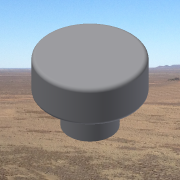
# Autodesk Inventor part: chimney
Saved by Autodesk Inventor 2014 SP1 (Build 180222100, 222)
## iProperties
Created: 2014-05-23
Part Number: chimney
Material: Generic
Document SubType Name: Modeling
Designer: Dave
Density: 1 g/cm^3
Appearance: Default
Author: Dave
Autodesk Inventor part; units mm, degrees
ref_plane "YZ Plane" through (0, 0, 0) normal (1, 0, 0) x (0, 1, 0)
ref_plane "XZ Plane" through (0, 0, 0) normal (0, 1, 0) x (-1, 0, 0)
ref_plane "XY Plane" through (0, 0, 0) normal (0, 0, 1) x (1, 0, 0)
sketch "Sketch1" plane through (0, 0, 0) normal (0, 1, 0) x (-1, 0, 0)
  circle A0 centre (0, 0) radius 127
  circle A1 centre (0, 0) radius 125.73
  dimension "d0" = 254
  dimension "d1" = 1.27
  constraints: 2 centre point, 1 coincident
  measures "d0" diameter of A0
  measures "d1" radial gap between concentric circles of A1 A0
extrude "Extrusion1" add sketch "Sketch1" along normal blind 203.2
sketch "Sketch2" plane through (0, 203.2, 0) normal (0, 1, 0) x (1, 0, 0)
  circle A0 centre (0, 0) radius 125.73 projected
  circle A1 centre (0, 0) radius 127 projected
  point P0 (0, 127)
  constraints: 1 vertical alignment, 1 other
ref_plane "Work Plane1" through (0, 203.2, -127) normal (0, 0, -1) x (-1, 0, 0)
sketch "Sketch3" plane through (0, 203.2, -127) normal (0, 0, -1) x (-1, 0, 0)
  line L0 (-6.3336, -31.75) -> (6.3664, -31.75)
  line L1 (6.3664, -31.75) -> (6.3664, -12.7)
  line L2 (6.3664, -12.7) -> (-6.3336, -12.7)
  line L3 (-6.3336, -12.7) -> (-6.3336, -31.75)
  line L4 (127, 0) -> (-127, 0) projected
  point P0 (0, -203.2)
  point P1 (0.0164, -12.7)
  dimension "d4" = 12.7
  dimension "d5" = 19.05
  dimension "d6" = 12.7
  constraints: 8 end point, 2 parallel, 1 horizontal, 1 midpoint, 1 perpendicular
  measures "d4" distance of L0.start L0.end
  measures "d5" distance of L2.end L0.start
  measures "d6" distance between parallel lines of L2 L4
extrude "Extrusion2" add sketch "Sketch3" along normal blind 1.27
sketch "Sketch4" plane through (0, 203.2, -128.27) normal (0, 0, -1) x (-1, 0, 0)
  line L0 (-6.3336, -31.75) -> (6.3664, -31.75) projected
  line L1 (6.3664, -31.75) -> (6.3664, -12.7) projected
  line L2 (-6.3336, -31.75) -> (6.3664, -31.75)
  line L3 (6.3664, -31.75) -> (6.3664, -30.48)
  line L4 (6.3664, -30.48) -> (-6.3336, -30.48)
  line L5 (-6.3336, -30.48) -> (-6.3336, -31.75)
  point P0 (0, -203.2)
  dimension "d9" = 1.27
  constraints: 8 end point, 2 parallel, 1 horizontal, 1 perpendicular, 1 point on line
  measures "d9" distance between parallel lines of L2 L4
extrude "Extrusion3" add sketch "Sketch4" along normal blind 101.6
pattern_circular "Circular Pattern1" count 3 over 360 about axis through (0, -10, 0) along (0, 1, 0) of "Extrusion2", "Extrusion3"
ref_plane "Work Plane2" through (0, 203.2, 0) normal (0, 0, -1) x (-1, 0, 0)
sketch "Sketch6" plane through (0, 203.2, 0) normal (0, 0, -1) x (-1, 0, 0)
  line L0 (-217.2385, -33.7501) -> (-230.8245, -33.7501)
  arc A0 (-249.8745, -14.7001) -> (-230.8245, -33.7501) centre (-230.8245, -14.7001) ccw
  line L1 (-249.8745, -14.7001) -> (-249.8745, 137.6999)
  line L2 (-249.8745, 61.4999) -> (-198.9713, 61.4999) construction
  arc A1 (-230.8245, 156.7499) -> (-249.8745, 137.6999) centre (-230.8245, 137.6999) ccw
  line L3 (0, 0) -> (0, 173.8895) construction
  line L4 (-230.8245, 156.7499) -> (0, 156.7499)
  line L5 (0, 158.0199) -> (-230.8245, 158.0199)
  arc A2 (-230.8245, 158.0199) -> (-251.1445, 137.6999) centre (-230.8245, 137.6999) ccw
  line L6 (-251.1445, 137.6999) -> (-251.1445, -14.7001)
  arc A3 (-251.1445, -14.7001) -> (-230.8245, -35.0201) centre (-230.8245, -14.7001) ccw
  line L7 (-230.8245, -35.0201) -> (-217.2385, -35.0201)
  line L8 (0, 156.7499) -> (0, 158.0199)
  line L9 (-217.2385, -35.0201) -> (-217.2385, -33.7501)
  point P0 (0, -203.2)
  dimension "d19" = 38.1
  dimension "d20" = 152.4
  dimension "d21" = 1.27
  constraints: 20 end point, 8 point on circle, 6 perpendicular, 4 centre point, 2 symmetric about line, 2 tangent, 1 horizontal, 1 midpoint, 1 parallel, 1 point on line, 5 other
  measures "d19" diameter of A0
  measures "d20" distance of L1.start L1.end
  measures "d21" distance between parallel lines of L4 L5
revolve "Revolution2" add sketch "Sketch6" angle 360 about axis through (0, 203.2, 0) along (0, 1, 0)
body "Solid1"
